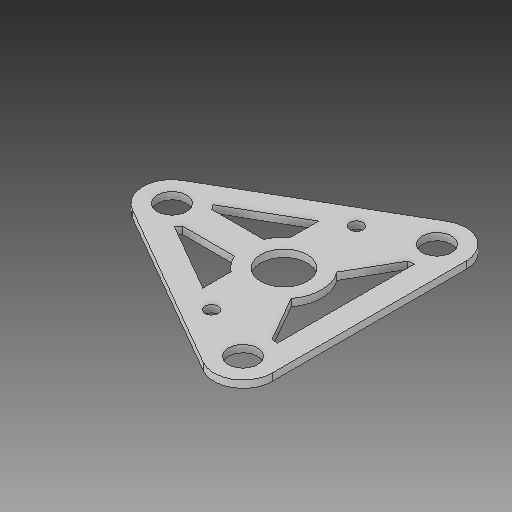
# Autodesk Inventor part: tri_headplate_2
Saved by Autodesk Inventor 2017 (Build 210142000, 142)
## iProperties
Created: 2017-03-20
Part Number: tri_headplate_2
Material: Generic
Document SubType Name: Modeling
Designer: richp
Density: 1 g/cm^3
Appearance: Default
bearing_edge_distance: 1.670 in
mounting_hole_distance: 1.248 in
Author: richp
Autodesk Inventor part; units mm, degrees
ref_plane "YZ Plane" through (0, 0, 0) normal (1, 0, 0) x (0, 1, 0)
ref_plane "XZ Plane" through (0, 0, 0) normal (0, 1, 0) x (-1, 0, 0)
ref_plane "XY Plane" through (0, 0, 0) normal (0, 0, 1) x (1, 0, 0)
sketch "Sketch1" plane through (0, 0, 0) normal (0, 1, 0) x (-1, 0, 0)
  circle A0 centre (0, 0) radius 5.08
  circle A1 centre (0, 0) radius 8.255 construction
  circle A2 centre (24.493, 0) radius 3.175
  line L0 (-23.8942, 0) -> (43.5551, 0) construction
  line L1 (0, 0) -> (-29.9334, 51.8461) construction
  line L2 (0, 0) -> (36.1069, 62.539) construction
  circle A3 centre (-12.2465, 21.2116) radius 3.175
  circle A4 centre (-12.2465, -21.2116) radius 3.175
  circle A5 centre (24.493, 0) radius 6.35 construction
  circle A6 centre (-12.2465, 21.2116) radius 6.35 construction
  circle A7 centre (-12.2465, -21.2116) radius 6.35 construction
  line L3 (18.9937, 3.175) -> (7.62, 3.175)
  line L4 (-12.2465, 14.8616) -> (-6.5596, 5.0116)
  line L5 (-12.2465, -14.8616) -> (-6.5596, -5.0116)
  line L6 (27.668, 5.4993) -> (-9.0715, 26.7108)
  line L7 (-18.5965, -21.2116) -> (-18.5965, 21.2116)
  line L8 (27.668, -5.4993) -> (-9.0715, -26.7108)
  arc A8 (27.668, -5.4993) -> (27.668, 5.4993) centre (24.493, 0) ccw
  arc A9 (-9.0715, 26.7108) -> (-18.5965, 21.2116) centre (-12.2465, 21.2116) ccw
  arc A10 (-18.5965, -21.2116) -> (-9.0715, -26.7108) centre (-12.2465, -21.2116) ccw
  line L9 (19.7398, 4.2107) -> (5.08, 12.6746)
  arc A11 (7.62, 3.175) -> (5.08, 6.5068) centre (0, 0) ccw
  arc A12 (19.7398, 4.2107) -> (18.9937, 3.175) centre (24.493, 0) ccw
  line L10 (18.9937, -3.175) -> (7.62, -3.175)
  line L11 (19.7398, -4.2107) -> (5.08, -12.6746)
  arc A13 (5.08, -6.5068) -> (7.62, -3.175) centre (0, 0) ccw
  arc A14 (18.9937, -3.175) -> (19.7398, -4.2107) centre (24.493, 0) ccw
  line L12 (-13.5165, 14.9899) -> (-13.5165, -14.9899)
  arc A15 (-13.5165, 14.9899) -> (-12.2465, 14.8616) centre (-12.2465, 21.2116) ccw
  arc A16 (-12.2465, -14.8616) -> (-13.5165, -14.9899) centre (-12.2465, -21.2116) ccw
  line L13 (5.08, 12.6746) -> (5.08, 6.5068)
  line L14 (5.08, -12.6746) -> (5.08, -6.5068)
  arc A17 (-6.5596, 5.0116) -> (-6.5596, -5.0116) centre (0, 0) ccw
  point P0 (0, 15.8496)
  dimension "d0" = 10.16
  dimension "d1" = 3.175
  dimension "d2" = 24.493
  dimension "d3" = 6.35
  dimension "d4" = 120
  dimension "d5" = 60
  dimension "d6" = 3.175
  dimension "d7" = 3.175
  dimension "d8" = 5.08
  dimension "d9" = 15.8496
  dimension "d10" = 24.493
  dimension "d12" = 3.175
  dimension "d13" = 5.08
  dimension "d14" = 5.08
  dimension "d30" = 21.209
  constraints: 30 end point, 30 point on circle, 17 centre point, 15 symmetric about line, 5 concentric, 5 tangent, 4 parallel, 3 coincident, 2 horizontal, 2 point on line, 1 vertical, 10 other
  measures "d0" diameter of A0
  measures "d1" radial gap between concentric circles of A0 A1
  measures "d2" distance of point (0, 0) A2.centre
  measures "d3" diameter of A2
  measures "d4" angle of L1 L0
  measures "d5" angle of L0 L2
  measures "d6" radial gap between concentric circles of A5 A2
  measures "d7" distance between parallel lines of L0 L3
  measures "d8" distance between parallel lines of L6 L9
  measures "d9" distance of point (0, 0) point (0, 15.85)
  measures "d10" horizontal distance of A2.centre point (0, 15.85)
  measures "d12" distance between parallel lines of L1 L4
  measures "d13" distance between parallel lines of L7 L12
  measures "d14" horizontal distance of L9.end point (0, 15.85)
extrude "Extrusion1" add sketch "Sketch1" against normal blind 1.5875
sketch "Sketch2" plane through (0, 0, 0) normal (0, 1, 0) x (1, 0, 0)
  line L0 (23.8942, 0) -> (-43.5551, 0) construction
  point P0 (0, 0)
  point P1 (0, -15.8496)
  point P2 (0, 15.8496)
  constraints: 1 symmetric about line
hole "Hole1" at (0, 0, 15.8496) at (0, 0, -15.8496) direction (0, -1, 0) diameter 2.8448 depth 25.4 tip angle 118
sketch "Sketch3" plane through (0, 0, 0) normal (0, 1, 0) x (1, 0, 0)
  circle A0 centre (0, -15.8496) radius 1.4224 projected
  circle A1 centre (0, 15.8496) radius 1.4224 projected
  arc A2 (6.5596, -5.0116) -> (6.5596, 5.0116) centre (0, 0) ccw projected
  line L0 (6.5596, 5.0116) -> (12.2465, 14.8616) projected
  arc A3 (12.2465, 14.8616) -> (13.5165, 14.9899) centre (12.2465, 21.2116) ccw projected
  line L1 (13.5165, 14.9899) -> (13.5165, -14.9899) projected
  arc A4 (13.5165, -14.9899) -> (12.2465, -14.8616) centre (12.2465, -21.2116) ccw projected
  line L2 (12.2465, -14.8616) -> (6.5596, -5.0116) projected
  circle A5 centre (0, 0) radius 5.08 projected
  arc A6 (-18.9937, 3.175) -> (-19.7398, 4.2107) centre (-24.493, 0) ccw projected
  line L3 (-19.7398, 4.2107) -> (-5.08, 12.6746) projected
  line L4 (-5.08, 12.6746) -> (-5.08, 6.5068) projected
  arc A7 (-5.08, 6.5068) -> (-7.62, 3.175) centre (0, 0) ccw projected
  line L5 (-7.62, 3.175) -> (-18.9937, 3.175) projected
  arc A8 (-19.7398, -4.2107) -> (-18.9937, -3.175) centre (-24.493, 0) ccw projected
  line L6 (-18.9937, -3.175) -> (-7.62, -3.175) projected
  arc A9 (-7.62, -3.175) -> (-5.08, -6.5068) centre (0, 0) ccw projected
  line L7 (-5.08, -6.5068) -> (-5.08, -12.6746) projected
  line L8 (-5.08, -12.6746) -> (-19.7398, -4.2107) projected
  circle A10 centre (12.2465, 21.2116) radius 3.175 projected
  circle A11 centre (12.2465, -21.2116) radius 3.175 projected
  circle A12 centre (-24.493, 0) radius 3.175 projected
  line L9 (-27.668, -5.4993) -> (9.0715, -26.7108) projected
  arc A13 (9.0715, -26.7108) -> (18.5965, -21.2116) centre (12.2465, -21.2116) ccw projected
  line L10 (18.5965, -21.2116) -> (18.5965, 21.2116) projected
  arc A14 (18.5965, 21.2116) -> (9.0715, 26.7108) centre (12.2465, 21.2116) ccw projected
  line L11 (9.0715, 26.7108) -> (-27.668, 5.4993) projected
  arc A15 (-27.668, 5.4993) -> (-27.668, -5.4993) centre (-24.493, 0) ccw projected
  line L12 (0, 0) -> (29.9334, -51.8461) construction
  line L13 (23.8942, 0) -> (-43.5551, 0) construction
  circle A16 centre (12.2465, -21.2116) radius 6.35 construction
  circle A17 centre (0, 0) radius 8.255 construction
  line L14 (6.5596, -5.0116) -> (12.2465, -14.8616) projected
  line L15 (6.5596, -5.0116) -> (12.2465, -14.8616)
  line L16 (9.0715, -15.7123) -> (4.1275, -7.149)
  arc A18 (12.2465, -14.8616) -> (9.0715, -15.7123) centre (12.2465, -21.2116) ccw
  arc A19 (4.1275, -7.149) -> (6.5596, -5.0116) centre (0, 0) ccw
  line L17 (12.2465, 14.8616) -> (6.5596, 5.0116)
  line L18 (9.0715, 15.7123) -> (4.1275, 7.149)
  arc A20 (9.0715, 15.7123) -> (12.2465, 14.8616) centre (12.2465, 21.2116) ccw
  arc A21 (6.5596, 5.0116) -> (4.1275, 7.149) centre (0, 0) ccw
  dimension "d24" = 3.175
  constraints: 9 point on circle, 8 end point, 4 centre point, 3 symmetric about line, 1 collinear, 1 concentric, 1 parallel, 5 other
  measures "d24" distance between parallel lines of L2 L16
extrude "Extrusion2" [suppressed]
chamfer "Chamfer1" [suppressed]
equation "\"d2\" = mount_radius"
equation "\"d4\" = tri_angle"
equation "\"d5\" = 0.5 * d4"
equation "\"d9\" = 0.5 * mounting_hole_distance"
equation "\"d13\" = d8"
equation "\"d15\" = material_thickness"
equation "\"d27\" = material_thickness"
equation "\"material_thickness\" = 1.5875"
equation "\"bearing_edge_distance\" = 2 * d30"
equation "\"tri_angle\" = 120deg"
equation "\"mount_radius\" = 24.493"
equation "\"mounting_hole_distance\" = 31.6992"
body "Solid1"
